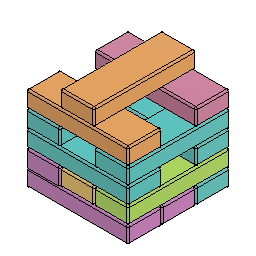
01-Default (Autodesk Fusion 360 design; units mm, degrees)
Autodesk Fusion 360 part; units mm, degrees
sketch "Sketch1" plane through (0, 0, 0) normal (0, 0, 1) x (1, 0, 0)
  line L0 (30, -10) -> (-30, -10)
  line L1 (-30, -10) -> (-30, 10)
  line L2 (-30, 10) -> (30, 10)
  line L3 (30, 10) -> (30, -10)
  line L4 (30, -10) -> (-30, 10) construction
  line L5 (-30, -10) -> (30, 10) construction
  dimension "d1" = 60
  dimension "d2" = 20
  constraint horizontal L0
  constraint perpendicular L0 L1
  constraint parallel L0 L2
  constraint parallel L1 L3
  constraint coincident L4 origin
  constraint coincident L5 origin
  measures "d1" distance of L1.end L2.end
  measures "d2" distance of L0.end L1.end
extrude "Extrude1" add sketch "Sketch1" along normal blind 10 makes body 1
copy_body "CopyPasteBodies1" bodies 1 makes body 2
move_body "Move1" bodies 2 to x (1, 0, 0) y (0, 1, 0) z (0, 0, 1) at (0, -20, 0)
copy_body "CopyPasteBodies2" bodies 1 makes body 3
move_body "Move2" bodies 3 to x (1, 0, 0) y (0, 1, 0) z (0, 0, 1) at (0, 20, 0)
copy_body "CopyPasteBodies3" bodies 1 makes body 4
move_body "Move3" bodies 4 to x (0, 1, 0) y (-1, 0, 0) z (0, 0, 1) at (-90, 0, 20)
move_body "Move4" bodies 4 to x (1, 0, 0) y (0, 1, 0) z (0, 0, 1) at (70, 0, -10)
sketch "Sketch1 (2)" plane through (0, 0, 0) normal (0, 0, 1) x (1, 0, 0) in component "blockExtrudedFromOffset"
  line L0 (10, 30) -> (-10, 30)
  line L1 (-10, 30) -> (-10, -30)
  line L2 (-10, -30) -> (10, -30)
  line L3 (10, -30) -> (10, 30)
  line L4 (10, 30) -> (-10, -30) construction
  line L5 (-10, 30) -> (10, -30) construction
  dimension "d9" = 20
  dimension "d10" = 60
  constraint horizontal L0
  constraint perpendicular L0 L1
  constraint parallel L0 L2
  constraint parallel L1 L3
  constraint coincident L4 origin
  constraint coincident L5 origin
  measures "d9" distance of L1.end L2.end
  measures "d10" distance of L0.end L1.end
extrude "Extrude1'" add sketch "Sketch1 (2)" along normal blind 10 from surface at 10 separate body makes body 5 in component "blockExtrudedFromOffset"
sketch "Sketch1 (3)" plane through (0, 0, 0) normal (0, 0, 1) x (1, 0, 0) in component "block"
  line L0 (-30, 10) -> (30, 10)
  line L1 (30, 10) -> (30, 30)
  line L2 (30, 30) -> (-30, 30)
  line L3 (-30, 30) -> (-30, 10)
  line L4 (-30, 10) -> (30, 30) construction
  line L5 (30, 10) -> (-30, 30) construction
  point P0 (30, 10)
  point P1 (0, 20)
  dimension "d14" = 20
  dimension "d15" = 60
  constraint horizontal L0
  constraint perpendicular L0 L1
  constraint parallel L0 L2
  constraint parallel L1 L3
  constraint coincident L4 P1
  constraint coincident L5 P1
  constraint coincident P0 L0.end
  measures "d14" distance of P0 L1.end
  measures "d15" distance of L1.end L2.end
extrude "Extrude1''" add sketch "Sketch1 (3)" along normal blind 10 separate body makes body 6 in component "block"
sketch "Sketch1 (4)" plane through (0, 0, 0) normal (0, 0, 1) x (1, 0, 0) in component "blockMovedBody"
  line L0 (-30, 10) -> (30, 10)
  line L1 (30, 10) -> (30, 30)
  line L2 (30, 30) -> (-30, 30)
  line L3 (-30, 30) -> (-30, 10)
  line L4 (-30, 10) -> (30, 30) construction
  line L5 (30, 10) -> (-30, 30) construction
  point P0 (30, 10)
  point P1 (0, 20)
  dimension "d14_1" = 20
  dimension "d15_1" = 60
  constraint horizontal L0
  constraint perpendicular L0 L1
  constraint parallel L0 L2
  constraint parallel L1 L3
  constraint coincident L4 P1
  constraint coincident L5 P1
  constraint coincident P0 L0.end
  measures "d14_1" distance of P0 L1.end
  measures "d15_1" distance of L1.end L2.end
extrude "Extrude1'''" add sketch "Sketch1 (4)" along normal blind 10 separate body makes body 7 in component "blockMovedBody"
move_body "Move1'" bodies 7 to x (0, -1, 0) y (1, 0, 0) z (0, 0, 1) at (0, 0, 10) in component "blockMovedBody"
sketch "Sketch1 (5)" plane through (0, 0, 0) normal (0, 0, 1) x (1, 0, 0) in component "mixed"
  line L0 (-30, 10) -> (30, 10)
  line L1 (30, 10) -> (30, 30)
  line L2 (30, 30) -> (-30, 30)
  line L3 (-30, 30) -> (-30, 10)
  line L4 (-30, 10) -> (30, 30) construction
  line L5 (30, 10) -> (-30, 30) construction
  point P0 (30, 10)
  point P1 (0, 20)
  dimension "d14_2" = 20
  dimension "d15_2" = 60
  constraint horizontal L0
  constraint perpendicular L0 L1
  constraint parallel L0 L2
  constraint parallel L1 L3
  constraint coincident L4 P1
  constraint coincident L5 P1
  constraint coincident P0 L0.end
  measures "d14_2" distance of P0 L1.end
  measures "d15_2" distance of L1.end L2.end
extrude "Extrude1''''" add sketch "Sketch1 (5)" along normal blind 10 separate body makes body 8 in component "mixed"
sketch "Sketch1 (6)" plane through (0, 0, 0) normal (0, 0, 1) x (1, 0, 0) in component "subComponentWithBodies"
  line L0 (-30, 10) -> (30, 10)
  line L1 (30, 10) -> (30, 30)
  line L2 (30, 30) -> (-30, 30)
  line L3 (-30, 30) -> (-30, 10)
  line L4 (-30, 10) -> (30, 30) construction
  line L5 (30, 10) -> (-30, 30) construction
  point P0 (30, 10)
  point P1 (0, 20)
  dimension "d14_3" = 20
  dimension "d15_3" = 60
  constraint horizontal L0
  constraint perpendicular L0 L1
  constraint parallel L0 L2
  constraint parallel L1 L3
  constraint coincident L4 P1
  constraint coincident L5 P1
  constraint coincident P0 L0.end
  measures "d14_3" distance of P0 L1.end
  measures "d15_3" distance of L1.end L2.end
extrude "Extrude1'''''" add sketch "Sketch1 (6)" along normal blind 10 separate body makes body 9 in component "subComponentWithBodies"
sketch "Sketch1 (7)" plane through (0, 0, 0) normal (0, 0, 1) x (1, 0, 0) in component "hiddenComponent"
  line L0 (-30, 10) -> (30, 10)
  line L1 (30, 10) -> (30, 30)
  line L2 (30, 30) -> (-30, 30)
  line L3 (-30, 30) -> (-30, 10)
  line L4 (-30, 10) -> (30, 30) construction
  line L5 (30, 10) -> (-30, 30) construction
  point P0 (30, 10)
  point P1 (0, 20)
  dimension "d14_4" = 20
  dimension "d15_4" = 60
  constraint horizontal L0
  constraint perpendicular L0 L1
  constraint parallel L0 L2
  constraint parallel L1 L3
  constraint coincident L4 P1
  constraint coincident L5 P1
  constraint coincident P0 L0.end
  measures "d14_4" distance of P0 L1.end
  measures "d15_4" distance of L1.end L2.end
extrude "Extrude1''''''" add sketch "Sketch1 (7)" along normal blind 10 separate body makes body 10 in component "hiddenComponent"
sketch "Sketch1 (8)" plane through (0, 0, 0) normal (0, 0, 1) x (1, 0, 0) in component "hiddenBodyFolder"
  line L0 (-30, 10) -> (30, 10)
  line L1 (30, 10) -> (30, 30)
  line L2 (30, 30) -> (-30, 30)
  line L3 (-30, 30) -> (-30, 10)
  line L4 (-30, 10) -> (30, 30) construction
  line L5 (30, 10) -> (-30, 30) construction
  point P0 (30, 10)
  point P1 (0, 20)
  dimension "d14_5" = 20
  dimension "d15_5" = 60
  constraint horizontal L0
  constraint perpendicular L0 L1
  constraint parallel L0 L2
  constraint parallel L1 L3
  constraint coincident L4 P1
  constraint coincident L5 P1
  constraint coincident P0 L0.end
  measures "d14_5" distance of P0 L1.end
  measures "d15_5" distance of L1.end L2.end
extrude "Extrude1'''''''" add sketch "Sketch1 (8)" along normal blind 10 separate body makes body 11 in component "hiddenBodyFolder"
sketch "Sketch1 (9)" plane through (0, 0, 0) normal (0, 0, 1) x (1, 0, 0) in component "hiddenBody"
  line L0 (-30, 10) -> (30, 10)
  line L1 (30, 10) -> (30, 30)
  line L2 (30, 30) -> (-30, 30)
  line L3 (-30, 30) -> (-30, 10)
  line L4 (-30, 10) -> (30, 30) construction
  line L5 (30, 10) -> (-30, 30) construction
  point P0 (30, 10)
  point P1 (0, 20)
  dimension "d14_6" = 20
  dimension "d15_6" = 60
  constraint horizontal L0
  constraint perpendicular L0 L1
  constraint parallel L0 L2
  constraint parallel L1 L3
  constraint coincident L4 P1
  constraint coincident L5 P1
  constraint coincident P0 L0.end
  measures "d14_6" distance of P0 L1.end
  measures "d15_6" distance of L1.end L2.end
extrude "Extrude1''''''''" add sketch "Sketch1 (9)" along normal blind 10 separate body makes body 12 in component "hiddenBody"
copy_body "CopyPasteBodies1'" bodies 9 makes body 13 in component "subComponentWithBodies"
move_body "Move1''" bodies 13 to x (0, 1, 0) y (-1, 0, 0) z (0, 0, 1) at (20, 40, 10) in component "subComponentWithBodies"
fillet "Fillet1" radius 1 4 faces at (-10, 10, 3.3333) (-10, 23.3333, 10) (10, 30, 3.3333) (-10, 23.3333, 0) on bodies 6 in component "block"
fillet "Fillet1'" radius 1 8 faces at (-10, 23.3333, 10) (10, 30, 3.3333) (-10, 10, 3.3333) (-10, 23.3333, 0) (3.3333, 30, 20) (10, 30, 13.3333) (-10, 50, 13.3333) (3.3333, 30, 10) on bodies 9 13 in component "subComponentWithBodies"
fillet "Fillet1''" radius 1 4 faces at (-3.3333, 10, 20) (-3.3333, 10, 10) (-10, 10, 13.3333) (10, -10, 13.3333) on bodies 5 in component "blockExtrudedFromOffset"
fillet "Fillet1'''" radius 1 4 faces at (16.6667, 10, 20) (10, 10, 13.3333) (30, -10, 13.3333) (16.6667, 10, 10) on bodies 7 in component "blockMovedBody"
fillet "Fillet1''''" radius 1 4 faces at (-10, 23.3333, 10) (-10, 23.3333, 0) (10, 30, 3.3333) (-10, 10, 3.3333) on bodies 8 in component "mixed"
fillet "Fillet1'''''" radius 1 11 faces at (10, -3.3333, 10) (10, -3.3333, 0) (-10, 10, 3.3333) (10, -10, 3.3333) (10, -23.3333, 10) (10, -30, 3.3333) (10, -23.3333, 0) (-10, -10, 3.3333) (-16.6667, 10, 20) (-30, -10, 13.3333) (-10, 10, 13.3333) on bodies 1 2 4
component "blockExtrudedFromOffset" placed x (1, 0, 0) y (0, 1, 0) z (0, 0, 1) at (0, 0, 0)
component "block" placed x (1, 0, 0) y (0, 1, 0) z (0, 0, 1) at (0, 0, 0)
component "block" placed x (1, 0, 0) y (0, 1, 0) z (0, 0, 1) at (0, 0, 20)
component "block" placed x (1, 0, 0) y (0, 1, 0) z (0, 0, 1) at (0, -40, 20)
component "blockMovedBody" placed x (1, 0, 0) y (0, 1, 0) z (0, 0, 1) at (0, 0, 0)
component "blocks" placed x (1, 0, 0) y (0, 1, 0) z (0, 0, 1) at (0, 0, 0)
component "block" placed x (0, -1, 0) y (1, 0, 0) z (0, 0, 1) at (-40, 0, 30) in component "blocks"
component "deep" placed x (1, 0, 0) y (0, 1, 0) z (0, 0, 1) at (0, 0, 0) in component "blocks"
component "mixed" placed x (1, 0, 0) y (0, 1, 0) z (0, 0, 1) at (0, 0, 40) in component "blocks"
component "hiddenComponent" placed x (0, -1, 0) y (1, 0, 0) z (0, 0, 1) at (-20, 0, 50) in component "blocks"
component "hiddenBodyFolder" placed x (0, -1, 0) y (1, 0, 0) z (0, 0, 1) at (0, 0, 50) in component "blocks"
component "hiddenBody" placed x (0, -1, 0) y (1, 0, 0) z (0, 0, 1) at (-40, 0, 50) in component "blocks"
component "deeper" placed x (1, 0, 0) y (0, 1, 0) z (0, 0, 1) at (0, 0, 0) in component "deep"
component "deepest" placed x (1, 0, 0) y (0, 1, 0) z (0, 0, 1) at (0, 0, 0) in component "deeper"
component "block" placed x (0, -1, 0) y (1, 0, 0) z (0, 0, 1) at (0, 0, 30) in component "deepest"
component "subComponentWithBodies" placed x (1, 0, 0) y (0, 1, 0) z (0, 0, 1) at (0, -40, 0) in component "mixed"
hidden bodies 3 12
named bodies: "rootBody", "copiedInPlaceBody", "hiddenBody", "copiedAndMovedafterwardsBody", "blockExtrudedFromOffset", "blockMovedBody", "bodyInComponentWithSubComponents", "hiddenComponent", "hiddenBodyFolder"
